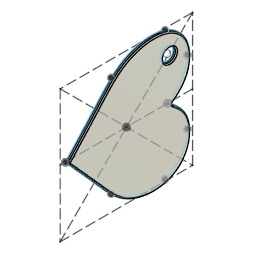
Srdce v3 (Autodesk Fusion 360 design; units mm, degrees)
Autodesk Fusion 360 part; units mm, degrees
sketch "Sketch1" plane through (0, 0, 0) normal (1, 0, 0) x (0, 1, 0)
  line L0 (25, 25) -> (-25, 25) construction
  line L1 (-25, 25) -> (-25, -25) construction
  line L2 (-25, -25) -> (25, -25) construction
  line L3 (25, -25) -> (25, 25) construction
  line L4 (25, 25) -> (-25, -25) construction
  line L5 (-25, 25) -> (25, -25) construction
  line L6 (25, 0) -> (-25, 0) construction
  spline S0 degree 5 poles (15.5332, 0) (16.1901, -0.3985) (17.4337, -1.233) (19.0878, -2.5973) (20.8692, -4.6424) (22.3741, -7.5604) (23.1291, -10.7838) (23.094, -14.1955) (22.2101, -17.5827) (20.4242, -20.6629) (17.7316, -23.1462) (14.211, -24.7854) (10.0736, -25.4363) (5.6864, -25.1034) (1.4565, -23.8906) (-2.2946, -21.9639) (-5.4026, -19.5107) (-8.0736, -16.7032) (-10.7572, -13.6579) (-13.5826, -10.4443) (-16.5999, -7.0972) (-19.1265, -4.3212) (-21.0554, -2.183) (-22.3507, -0.7319) (-23.0007, 0) knots 0 0 0 0 0 0 0.05 0.1 0.15 0.2 0.25 0.3 0.35 0.4 0.45 0.5 0.55 0.6 0.65 0.7 0.75 0.8 0.85 0.9 0.95 1 1 1 1 1 1
  line L7 (-18.5016, -5.066) -> (-27.4998, 5.066)
  line L8 (-1.736, -22.7654) -> (-9.8005, -15.2102)
  spline S1 degree 5 poles (15.5332, 0) (16.1901, 0.3985) (17.4337, 1.233) (19.0878, 2.5973) (20.8692, 4.6424) (22.3741, 7.5604) (23.1291, 10.7838) (23.094, 14.1955) (22.2101, 17.5827) (20.4242, 20.6629) (17.7316, 23.1462) (14.211, 24.7854) (10.0736, 25.4363) (5.6864, 25.1034) (1.4565, 23.8906) (-2.2946, 21.9639) (-5.4026, 19.5107) (-8.0736, 16.7032) (-10.7572, 13.6579) (-13.5826, 10.4443) (-16.5999, 7.0972) (-19.1265, 4.3212) (-21.0554, 2.183) (-22.3507, 0.7319) (-23.0007, 0) knots 0 0 0 0 0 0 0.05 0.1 0.15 0.2 0.25 0.3 0.35 0.4 0.45 0.5 0.55 0.6 0.65 0.7 0.75 0.8 0.85 0.9 0.95 1 1 1 1 1 1
  line L9 (9.6982, 3.5392) -> (21.3682, -3.5392)
  line L10 (9.6982, -3.5392) -> (21.3682, 3.5392)
  line L11 (-1.736, 22.7654) -> (-9.8005, 15.2102)
  line L12 (-18.5016, 5.066) -> (-27.4998, -5.066)
  circle A0 centre (15.2067, 16.4096) radius 2.5
  point P0 (23.0091, -12.1118)
  point P1 (14.5627, -24.3783)
  point P2 (-5.7683, -18.9878)
  point P3 (23.0091, 12.1118)
  point P4 (14.5627, 24.3783)
  point P5 (-5.7683, 18.9878)
  dimension "d1" = 50
  dimension "d2" = 50
  dimension "d15" = 5
  constraint horizontal L0
  constraint perpendicular L0 L1
  constraint parallel L0 L2
  constraint parallel L1 L3
  constraint coincident L4 origin
  constraint coincident L5 origin
  constraint midpoint L3 L6.start
  constraint midpoint L1 L6.end
  constraint coincident L6 S0.start
  constraint coincident L6 S0.end
  constraint midpoint S0.end L7
  constraint midpoint P2 L8
  constraint midpoint S0.start L9
  constraint symmetric L6 S0.start S1.start
  constraint symmetric L6 P0 P3
  constraint symmetric L6 P1 P4
  constraint symmetric L6 P2 P5
  constraint symmetric L6 S0.end S1.end
  constraint symmetric L6 L7.start L12.start
  constraint symmetric L6 L7.end L12.end
  constraint symmetric L6 L8.start L11.start
  constraint symmetric L6 L8.end L11.end
  constraint symmetric L6 L9.start L10.start
  constraint symmetric L6 L9.end L10.end
  measures "d1" distance of L1.end L2.end
  measures "d2" distance of L0.end L1.end
  measures "d15" diameter of A0
extrude "Extrude1" add sketch "Sketch1" along normal blind 1.2
fillet "Fillet1" radius 0.8 1 edges at (0.6, 15.5332, 0)
fillet "Fillet1" radius 0.5 1 edges at (0.6, -23.0007, 0)
chamfer "Chamfer2" distance 0.4 angle 45 1 faces at (1.2, -3.7558, -0.0076)
chamfer "Chamfer2" distance 0.2 angle 45 1 faces at (0, -3.7558, -0.0076)
named bodies: "Srdce"
